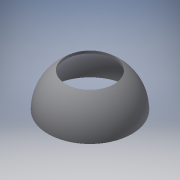
# Autodesk Inventor part: SentiBot top
Saved by Autodesk Inventor 2016 (Build 200138000, 138)
## iProperties
Created: 2015-07-02
Part Number: SentiBot top
Material: Generic
Document SubType Name: Modeling
Designer: Sudhar
Density: 1 g/cm^3
Appearance: Default
Author: Sudhar
Autodesk Inventor part; units mm, degrees
sketch "Sketch1" plane through (0, 0, 0) normal (0, 0, 1) x (1, 0, 0)
  arc A0 (21.6438, 2.6591) -> (-3.7562, 28.0591) centre (-3.7562, 2.6591) ccw
  line L0 (-3.7562, 28.0591) -> (-3.7562, 2.6591)
  line L1 (-3.7562, 2.6591) -> (22.0131, 2.6591)
  dimension "d0" = 50.8
  constraints: 4 end point, 2 point on circle, 1 centre point, 1 perpendicular, 1 point on line, 1 vertical
  measures "d0" diameter of A0
revolve "Revolution1" add sketch "Sketch1" angle 360 about axis through (-3.7562, 28.0591, 0) along (0, -1, 0)
ref_plane "Work Plane1" through (0, 0, 19.05) normal (0, 0, 1) x (1, 0, 0)
sketch "Sketch3" plane through (0, 0, 0) normal (0, 0, 1) x (1, 0, 0)
  line L0 (-3.675, 51.7812) -> (-3.675, -20.9618)
  constraints: 2 end point, 1 vertical
shell "Shell2" thickness 1.27 removed faces 1 at (1.2995, 2.6591, -4.9417)
ref_plane "Work Plane3" through (-11.1125, 0, 0) normal (1, 0, 0) x (0, 1, 0)
ref_plane "Work Plane5" through (-3.7562, 28.0591, 0) normal (0, 1, 0) x (-1, 0, 0)
sketch "Sketch12" plane through (-3.7562, 28.0591, 0) normal (0, 1, 0) x (-1, 0, 0)
  circle A0 centre (0, 0) radius 14.605
  dimension "d36" = 29.21
  constraints: 1 centre point
  measures "d36" diameter of A0
extrude "Extrusion8" cut sketch "Sketch12" against normal blind 25.4
body "Solid1"
